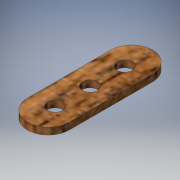
# Autodesk Inventor part: Top Panel
Saved by Autodesk Inventor 2016 SP2 (Build 200236200, 236)
## iProperties
Created: 2017-10-06
Part Number: Top Panel
Material: Generic
Document SubType Name: Modeling
Designer: Jared
Density: 1 g/cm^3
Appearance: White Ash - Java
Author: Jared
Autodesk Inventor part; units mm, degrees
ref_plane "YZ Plane" through (0, 0, 0) normal (1, 0, 0) x (0, 1, 0)
ref_plane "XZ Plane" through (0, 0, 0) normal (0, 1, 0) x (-1, 0, 0)
ref_plane "XY Plane" through (0, 0, 0) normal (0, 0, 1) x (1, 0, 0)
sketch "Sketch1" plane through (0, 0, 0) normal (0, 1, 0) x (-1, 0, 0)
  line L0 (0, -38.1) -> (0, 38.1) construction
  line L1 (19.05, -38.1) -> (19.05, 38.1)
  line L2 (-19.05, 38.1) -> (-19.05, -38.1)
  arc A0 (-19.05, -38.1) -> (19.05, -38.1) centre (0, -38.1) ccw
  arc A1 (19.05, 38.1) -> (-19.05, 38.1) centre (0, 38.1) ccw
  circle A2 centre (0, 0) radius 6.985
  circle A3 centre (0, -31.75) radius 6.985
  circle A4 centre (0, 31.75) radius 6.985
  line L3 (34.1256, 57.15) -> (-20.0171, 57.15)
  line L4 (24.6444, -57.15) -> (-26.3115, -57.15)
  dimension "d0" = 38.1
  dimension "d1" = 38.1
  dimension "d2" = 13.97
  dimension "d3" = 31.75
  dimension "d4" = 31.75
  dimension "d7" = 114.3
  constraints: 12 end point, 6 tangent, 5 centre point, 4 point on circle, 2 equal radius, 2 perpendicular, 1 coincident, 1 midpoint, 1 parallel, 1 point on line, 1 vertical
  measures "d0" distance of point (0, 0) L0.end
  measures "d1" diameter of A1
  measures "d2" diameter of A2
  measures "d3" distance of A2.centre A4.centre
  measures "d4" distance of A3.centre point (0, 0)
  measures "d7" distance between parallel lines of L4 L3
extrude "Extrusion1" add sketch "Sketch1" along normal blind 6.35
body "Solid1"
